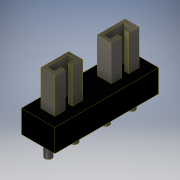
# Autodesk Inventor part: BK-6013_MiniATC_Fuse_Holder
Saved by Autodesk Inventor 2016 (Build 200138000, 138)
## iProperties
Created: 2016-09-30
Part Number: BK-6013_MiniATC_Fuse_Holder
Material: Generic
Document SubType Name: Modeling
Designer: jfixelle
Density: 1 g/cm^3
Appearance: Silver
Author: jfixelle
Autodesk Inventor part; units mm, degrees
ref_plane "YZ Plane" through (0, 0, 0) normal (1, 0, 0) x (0, 1, 0)
ref_plane "XZ Plane" through (0, 0, 0) normal (0, 1, 0) x (-1, 0, 0)
ref_plane "XY Plane" through (0, 0, 0) normal (0, 0, 1) x (1, 0, 0)
sketch "Sketch1" plane through (0, 0, 0) normal (0, 1, 0) x (-1, 0, 0)
  line L0 (2.375, 7.35) -> (-2.375, 7.35)
  line L1 (-2.375, 7.35) -> (-2.375, -7.35)
  line L2 (-2.375, -7.35) -> (2.375, -7.35)
  line L3 (2.375, -7.35) -> (2.375, 7.35)
  point P0 (0, 0)
  dimension "d0" = 14.7
  dimension "d1" = 4.75
  dimension "d2" = 2.375
  dimension "d3" = 7.35
  constraints: 8 end point, 2 parallel, 1 horizontal, 1 perpendicular
  measures "d0" distance of L2.end L0.start
  measures "d1" distance of L1.end L2.end
  measures "d2" distance from line of point (0, 0) L3
  measures "d3" distance from line of point (0, 0) L2
extrude "Extrusion1" add sketch "Sketch1" along normal blind 3.2
sketch "Sketch2" plane through (0, 0, 0) normal (0, -1, 0) x (1, 0, 0)
  circle A0 centre (0, 5.895) radius 0.5
  circle A1 centre (0, 2.235) radius 0.5
  point P0 (0, 0)
  dimension "d6" = 3.66
  dimension "d7" = 2.235
  dimension "d8" = 1
  dimension "d9" = 1
  constraints: 2 centre point
  measures "d6" distance of A1.centre A0.centre
  measures "d7" distance of point (0, 0) A1.centre
  measures "d8" diameter of A0
  measures "d9" diameter of A1
extrude "Extrusion2" add sketch "Sketch2" along normal blind 2.3
sketch "Sketch3" plane through (0, 3.2, 0) normal (0, 1, 0) x (1, 0, 0)
  line L0 (-1, -5.98) -> (1, -5.98)
  line L1 (1, -5.98) -> (1, -2.02)
  line L2 (1, -2.02) -> (-1, -2.02)
  line L3 (-1, -2.02) -> (-1, -5.98)
  line L4 (-1, -4) -> (1, -4) construction
  line L5 (-0.6, -5.45) -> (0.4, -5.45)
  line L6 (0.4, -5.45) -> (0.4, -2.4349)
  line L7 (0.4, -2.4349) -> (-0.6, -2.4349)
  line L8 (-0.6, -2.4349) -> (-0.6, -5.45)
  line L9 (0.4, -4.5) -> (1, -4.5)
  line L10 (1, -4.5) -> (1, -3.5)
  line L11 (1, -3.5) -> (0.4, -3.5)
  line L12 (0.4, -3.5) -> (0.4, -4.5)
  point P0 (0, 0)
  dimension "d12" = 4
  dimension "d13" = 3.96
  dimension "d14" = 1
  dimension "d15" = 0.4
  dimension "d16" = 5.45
  dimension "d17" = 3.0151
  dimension "d18" = 2
  dimension "d19" = 1
  dimension "d20" = 0.5
  dimension "d21" = 1
  constraints: 26 end point, 6 parallel, 3 horizontal, 3 perpendicular, 2 midpoint, 2 point on line
  measures "d12" distance from line of point (0, 0) L4
  measures "d13" distance of L2.end L0.start
  measures "d14" distance of L5.start L5.end
  measures "d15" distance between parallel lines of L3 L8
  measures "d16" distance from line of point (0, 0) L5
  measures "d17" distance of L5.end L6.end
  measures "d18" distance of L1.end L2.end
  measures "d19" distance from line of point (0, 0) L3
  measures "d20" distance between parallel lines of L4 L11
  measures "d21" distance between parallel lines of L9 L11
extrude "Extrusion3" add sketch "Sketch3" along normal blind 5 contours L3 L2 L1 L11 L6 L7 L8 L5 L9 L0
mirror "Mirror1" about plane through (0, 0, 0) normal (0, 0, 1) of "Extrusion3", "Extrusion2"
body "Solid1"
